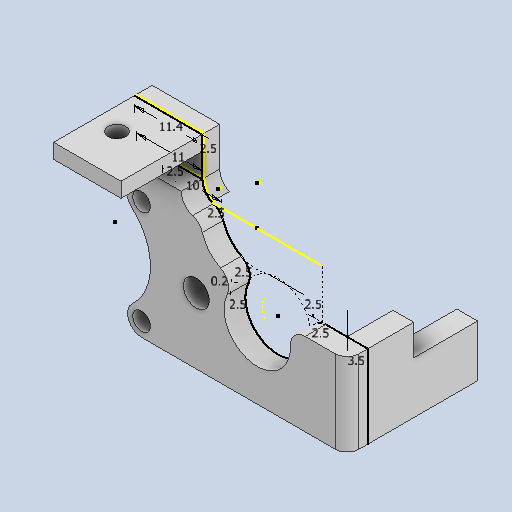
# Autodesk Inventor part: MotorEncoderBracket
Saved by Autodesk Inventor 2022 (Build 260153070, 153G)
## iProperties
Created: 2021-11-27
Part Number: MotorEncoderBracket
Material: Generic
Document SubType Name: Modeling
Designer: a laptop
Density: 1 g/cm^3
Appearance: Default
Author: a laptop
Autodesk Inventor part; units mm, degrees
ref_plane "YZ Plane" through (0, 0, 0) normal (1, 0, 0) x (0, 1, 0)
ref_plane "XZ Plane" through (0, 0, 0) normal (0, 1, 0) x (-1, 0, 0)
ref_plane "XY Plane" through (0, 0, 0) normal (0, 0, 1) x (1, 0, 0)
sketch "Sketch1" plane through (0, 0, 0) normal (0, 0, 1) x (1, 0, 0)
  circle A0 centre (-13, 8.75) radius 1.5 projected
  circle A1 centre (-3.75, 0) radius 2 construction
  circle A2 centre (-13, -8.75) radius 1.5 projected
  arc A3 (4.5834, 1.85) -> (4.5834, -1.85) centre (6.55, 0) ccw construction
  arc A4 (4.8736, 5.3432) -> (1.4897, 2.3987) centre (6.55, 0) ccw construction
  circle A5 centre (-3.75, 0) radius 2.2
  arc A6 (-14.5962, -6.9913) -> (-14.5962, 6.9913) centre (-20.9415, 0) ccw
  arc A7 (-13, 11.125) -> (-15.0744, 7.5935) centre (-13, 8.75) ccw construction
  line L0 (14.125, 11.125) -> (-18.25, 11.125) projected
  line L1 (-18.25, -11.125) -> (14.125, -11.125) projected
  arc A8 (-14.5962, -6.9913) -> (-13, -11.125) centre (-13, -8.75) ccw
  line L2 (-11.5, 8.75) -> (-11.5, -8.75) construction
  line L3 (21.75, 2.8432) -> (21.75, -11.125)
  line L4 (21.75, -11.125) -> (14.125, -11.125)
  line L5 (14.125, -11.125) -> (14.125, 11.125) construction
  line L6 (18.25, -7) -> (18.25, 7) construction
  arc A9 (-3, 11.125) -> (-2.7358, 9.3552) centre (3.0597, 11.125) ccw construction
  arc A10 (-2.7358, 9.3552) -> (-4.3762, 11.0097) centre (-5.1268, 8.625) ccw
  arc A11 (-2.7358, 9.3552) -> (0.349, 5.7054) centre (3.0597, 11.125) ccw
  line L7 (11.3745, 2.8432) -> (14.6427, 2.8432) construction
  arc A12 (11.3745, 2.8432) -> (4.8736, 5.3432) centre (6.55, 0) ccw construction
  arc A13 (1.4897, 2.3987) -> (0.349, 5.7054) centre (-0.7693, 3.4695) ccw
  arc A14 (0.349, 5.7054) -> (4.8736, 5.3432) centre (3.0597, 11.125) ccw construction
  arc A15 (1.4897, 2.3987) -> (12.145, 0.2373) centre (6.55, 0) ccw
  arc A16 (14.6427, 2.8432) -> (12.145, 0.2373) centre (14.6427, 0.3432) ccw
  arc A17 (12.145, 0.2373) -> (11.3745, 2.8432) centre (6.55, 0) ccw construction
  line L8 (14.6427, 2.8432) -> (21.75, 2.8432)
  line L9 (-12.425, 16.375) -> (-15.425, 16.375) projected
  line L10 (-15.425, 17.675) -> (-12.425, 17.675) projected
  line L11 (-15.425, 17.675) -> (-17.6949, 17.675)
  line L12 (-12.425, 17.675) -> (-6.2949, 17.675)
  line L13 (-6.2949, 17.675) -> (-6.2949, 20.175)
  line L14 (-6.2949, 20.175) -> (-17.6949, 20.175)
  line L15 (-17.6949, 20.175) -> (-17.6949, 17.675)
  arc A18 (-17.6949, 17.675) -> (-15.0744, 7.5935) centre (3.0083, 17.675) ccw
  line L16 (-6.2949, 13.625) -> (-17.2949, 13.625)
  line L17 (-6.2949, 13.625) -> (-6.2949, 17.675)
  arc A19 (-6.2949, 13.625) -> (-4.3762, 11.0097) centre (-3.553, 13.625) ccw
  arc A20 (-4.3762, 11.0097) -> (-5.1268, 11.125) centre (-5.1268, 8.625) ccw construction
  arc A21 (-15.0744, 7.5935) -> (-14.5962, 6.9913) centre (-13, 8.75) ccw
  point P0 (0, 0)
  point P1 (-4.6789, 11.125)
  point P2 (-16.6314, 11.125)
  dimension "d0" = 0.2
  dimension "d1" = 2.5
  dimension "d3" = 3.5
  dimension "d4" = 10
  dimension "d5" = 2.5
  dimension "d6" = 2.5
  dimension "d7" = 2.5
  dimension "d8" = 2.5
  dimension "d16" = 2.5
  dimension "d17" = 2.5
  dimension "d18" = 11
  dimension "d19" = 11.4
  constraints: 37 point on circle, 26 end point, 19 tangent, 18 centre point, 7 perpendicular, 6 point on line, 3 horizontal, 3 horizontal alignment, 3 line through centre, 2 concentric, 1 parallel, 1 vertical, 1 vertical alignment, 4 other
  measures "d0" radial gap between concentric circles of A1 A5
  measures "d3" distance between parallel lines of L3 L6
  measures "d4" distance of A9.start A7.start
  measures "d5" radius of A10
  measures "d6" vertical distance of L7.start A4.start
  measures "d7" radius of A13
  measures "d8" radius of A16
  measures "d16" distance between parallel lines of L16 L0
  measures "d17" distance of L12.end L13.end
  measures "d18" distance of L16.start L16.end
  measures "d19" distance of L12.end L11.end
extrude "Extrusion1" add sketch "Sketch1" along normal blind 3.5 contours A6 A21 A18 L0 A19 A10 A11 A13 A15 A16 L8 L3 L4 L1 A8 | A18 L16 A19 L0
sketch "Sketch2" plane through (0, 0, 0) normal (0, 0, -1) x (-1, 0, 0)
  line L0 (-18.25, 7) -> (-18.25, -7) projected
  line L1 (-21.75, -11.125) -> (-21.75, 2.8432) projected
  line L2 (-18.25, -7) -> (-18.25, -11.125)
  line L3 (13, -11.125) -> (-21.75, -11.125) projected
  line L4 (-18.25, -11.125) -> (-21.75, -11.125)
  line L5 (-21.75, 2.8432) -> (-14.6427, 2.8432) projected
  line L6 (-21.75, 2.8432) -> (-18.25, 2.8432)
  point P0 (0, 0)
  constraints: 6 end point, 3 point on line, 1 horizontal, 1 vertical
extrude "Extrusion2" add sketch "Sketch2" along normal blind 18.55
fillet "Fillet1" radius 2 1 edges at (21.75, -4.1409, 3.5)
extrude "Extrusion3" add sketch "Sketch1" against normal blind 0.325 contours A18 L16 A19 L0
sketch "Sketch5" plane through (0, 0, -0.325) normal (0, 0, -1) x (-1, 0, 0)
  line L0 (17.2949, 13.625) -> (6.2949, 13.625) projected
  arc A0 (4.6789, 11.125) -> (6.2949, 13.625) centre (3.553, 13.625) ccw projected
  line L1 (4.6789, 11.125) -> (16.6314, 11.125) projected
  arc A1 (16.6314, 11.125) -> (17.2949, 13.625) centre (-3.0083, 17.675) ccw projected
  line L2 (6.2949, 13.625) -> (6.2949, 17.675) projected
  line L3 (6.2949, 17.675) -> (6.2949, 20.175) projected
  line L4 (6.2949, 20.175) -> (17.6949, 20.175) projected
  line L5 (17.6949, 20.175) -> (17.6949, 17.675) projected
  line L6 (12.425, 17.675) -> (6.2949, 17.675) projected
  line L7 (15.425, 17.675) -> (12.425, 17.675) projected
  line L8 (15.425, 17.675) -> (17.6949, 17.675) projected
  arc A2 (15.0744, 7.5935) -> (17.6949, 17.675) centre (-3.0083, 17.675) ccw projected
  line L9 (6.2949, 13.625) -> (17.2949, 13.625) projected
  point P0 (0, 0)
extrude "Extrusion4" add sketch "Sketch5" along normal blind 2.675
extrude "Extrusion5" add sketch "Sketch5" against normal blind 14 contours L8 L7 L6 L3 L4 L5
sketch "Sketch6" plane through (-17.6949, 17.675, -0.325) normal (0, -1, 0) x (1, 0, 0)
  circle A0 centre (3.7699, 7.075) radius 1.5 projected
  point P0 (17.6949, 0.325)
extrude "Extrusion6" cut sketch "Sketch6" against normal blind 14
sketch "Sketch7" plane through (21.75, -11.125, -18.55) normal (1, 0, 0) x (0, 0, -1)
  line L0 (-10.8, 13.75) -> (-10.8, 8.75) projected
  line L1 (-10.8, 13.75) -> (-10.8, 13.9682)
  line L2 (-18.55, 13.9682) -> (0, 13.9682) projected
  line L3 (-10.8, 8.75) -> (0, 8.75)
  line L4 (0, 0) -> (0, 13.9682) projected
  line L5 (0, 8.75) -> (0, 13.9682)
  point P0 (-18.55, 11.125)
  constraints: 6 end point, 1 collinear, 1 parallel, 1 point on line, 1 vertical
extrude "Extrusion7" cut sketch "Sketch7" against normal blind 10
body "Solid1"
